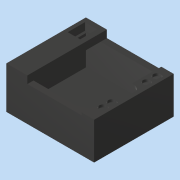
# Autodesk Inventor part: body
Saved by Autodesk Inventor 2017 (Build 210142000, 142)
## iProperties
Created: 2017-01-26
Part Number: body
Material: ABS Plastic
Document SubType Name: Modeling
Designer: techn
Density: 1.06 g/cm^3
Appearance: Smooth - Black
Author: techn
Autodesk Inventor part; units mm, degrees
ref_plane "YZ Plane" through (0, 0, 0) normal (1, 0, 0) x (0, 1, 0)
ref_plane "XZ Plane" through (0, 0, 0) normal (0, 1, 0) x (-1, 0, 0)
ref_plane "XY Plane" through (0, 0, 0) normal (0, 0, 1) x (1, 0, 0)
sketch "Sketch1" plane through (0, 0, 0) normal (0, 1, 0) x (-1, 0, 0)
  line L0 (0, 0) -> (35.5, 0)
  line L1 (35.5, 0) -> (35.5, -32.18)
  line L2 (35.5, -32.18) -> (0, -32.18)
  line L3 (0, -32.18) -> (0, 0)
  line L4 (33, -2.5) -> (2.5, -2.5)
  line L5 (2.5, -2.5) -> (2.5, -29.68)
  line L6 (2.5, -29.68) -> (33, -29.68)
  line L7 (33, -29.68) -> (33, -2.5)
  dimension "d0" = 32.18
  dimension "d1" = 35.5
  dimension "d2" = 2.5
  dimension "d3" = 2.5
  dimension "d4" = 2.5
  dimension "d5" = 2.5
  constraints: 16 end point, 4 parallel, 2 horizontal, 2 perpendicular
  measures "d0" distance of L2.end L0.start
  measures "d1" distance of L1.end L2.end
  measures "d2" distance between parallel lines of L1 L7
  measures "d3" distance between parallel lines of L0 L4
  measures "d4" distance between parallel lines of L3 L5
  measures "d5" distance between parallel lines of L2 L6
extrude "Extrusion1" add sketch "Sketch1" along normal blind 2 contours L0 L1 L2 L3 | L7 L6 L5 L4
extrude "Extrusion2" add sketch "Sketch1" along normal blind 14
sketch "Sketch2" plane through (0, 14, 0) normal (0, 1, 0) x (1, 0, 0)
  line L0 (-33, 2.5) -> (-33, 29.68) projected
  line L1 (-33, 29.68) -> (-2.5, 29.68) projected
  line L2 (-2.5, 29.68) -> (-2.5, 2.5) projected
  line L3 (-2.5, 2.5) -> (-33, 2.5) projected
  line L4 (-35.5, 0) -> (0, 0) projected
  line L5 (0, 0) -> (0, 32.18) projected
  line L6 (0, 32.18) -> (-35.5, 32.18) projected
  line L7 (-35.5, 32.18) -> (-35.5, 0) projected
  line L8 (-35.5, 0) -> (-35.5, 32.18) projected
  line L9 (0, 32.18) -> (-35.5, 32.18) projected
  line L10 (-35.5, 0) -> (-27, 0)
  line L11 (-27, 0) -> (-27, 32.18)
  line L12 (-27, 32.18) -> (-35.5, 32.18)
  line L13 (-35.5, 32.18) -> (-35.5, 0)
  dimension "d10" = 8.5
  constraints: 8 end point, 2 parallel, 1 horizontal, 1 perpendicular, 1 point on line
  measures "d10" distance between parallel lines of L7 L11
extrude "Extrusion3" add sketch "Sketch2" along normal blind 3 contours L3 L11 L4 L7 L6 L1 L0 | L0 L1 L11 L3
sketch "Sketch3" plane through (0, 17, 0) normal (0, 1, 0) x (1, 0, 0)
  line L0 (-35.5, 0) -> (-27, 0) projected
  line L1 (-27, 0) -> (-27, 32.18) projected
  line L2 (-27, 32.18) -> (-35.5, 32.18) projected
  line L3 (-35.5, 32.18) -> (-35.5, 0) projected
  line L4 (-34, 23.341) -> (-29, 23.341)
  line L5 (-29, 23.341) -> (-29, 30.341)
  line L6 (-29, 30.341) -> (-34, 30.341)
  line L7 (-34, 30.341) -> (-34, 23.341)
  point P0 (0, 0)
  dimension "d13" = 7
  dimension "d14" = 5
  dimension "d15" = 2
  constraints: 8 end point, 2 parallel, 1 horizontal, 1 perpendicular
  measures "d13" distance between parallel lines of L6 L4
  measures "d14" distance between parallel lines of L5 L7
  measures "d15" distance between parallel lines of L1 L5
extrude "Extrusion4" cut sketch "Sketch3" against normal blind 3 contours L7 L6 L5 L4
sketch "Sketch4" plane through (0, 14, 0) normal (0, 1, 0) x (1, 0, 0)
  line L0 (-27, 32.18) -> (-27, 29.68) projected
  line L1 (-27, 29.68) -> (-2.5, 29.68) projected
  line L2 (-2.5, 29.68) -> (-2.5, 2.5) projected
  line L3 (-2.5, 2.5) -> (-27, 2.5) projected
  line L4 (-27, 2.5) -> (-27, 0) projected
  line L5 (-27, 0) -> (0, 0) projected
  line L6 (0, 0) -> (0, 32.18) projected
  line L7 (0, 32.18) -> (-27, 32.18) projected
  line L8 (0, 32.18) -> (0, 0) projected
  line L9 (0, 0) -> (-35.5, 0) projected
  line L10 (0, 32.18) -> (-5, 32.18)
  line L11 (-5, 32.18) -> (-5, 0)
  line L12 (-5, 0) -> (0, 0)
  line L13 (0, 0) -> (0, 32.18)
  dimension "d18" = 5
  constraints: 8 end point, 2 parallel, 1 horizontal, 1 perpendicular, 1 point on line
  measures "d18" distance of L12.end L11.end
extrude "Extrusion5" add sketch "Sketch4" along normal blind 1 contours L7 L6 L5 L11 L3 L2 L1 | L1 L2 L3 L11
sketch "Sketch5" plane through (0, 15, 0) normal (0, 1, 0) x (1, 0, 0)
  line L0 (-5, 32.18) -> (-5, 0) projected
  line L1 (-5, 2.5) -> (-27, 2.5) projected
  line L2 (-5, 29.68) -> (-5, 2.5) projected
  circle A0 centre (-5, 16.5) radius 4
  line L3 (-2.5, 29.68) -> (-2.5, 2.5) projected
  circle A1 centre (-2.5, 27.937) radius 1.5
  circle A2 centre (-2.5, 23.7147) radius 1.5
  circle A3 centre (-2.5, 9.7184) radius 1.5
  circle A4 centre (-2.5, 6.1216) radius 1.5
  point P0 (0, 0)
  dimension "d21" = 8
  dimension "d22" = 14
  dimension "d23" = 3
  dimension "d24" = 3
  dimension "d25" = 3
  dimension "d26" = 3
  constraints: 5 centre point, 5 point on line
  measures "d21" diameter of A0
  measures "d22" distance of L1.start A0.centre
  measures "d23" diameter of A1
  measures "d24" diameter of A2
  measures "d25" diameter of A3
  measures "d26" diameter of A4
extrude "Extrusion6" cut sketch "Sketch5" against normal blind 1
equation "\"d3\" = d2"
equation "\"d4\" = d2"
equation "\"d5\" = d2"
body "Solid1"
